Autodesk Inventor part; units mm, degrees
(part 2 of 2)
sketch "Skizze29" plane through (89.6, -2.4765, -33.8) normal (0, 0, -1) x (-1, 0, 0)
  line L0 (43.6, -0.4235) -> (43.6, -0.5235) construction
  line L1 (43.6, -0.5235) -> (49.9, -0.5235) construction
  line L2 (49.9, -0.5235) -> (52.9, 2.4765) construction
  line L3 (52.9, 2.4765) -> (79.4, 2.4765) construction
  line L4 (79.4, 2.4765) -> (79.4, 2.2765) construction
  line L5 (79.4, 2.2765) -> (83.4, 2.2765) construction
  line L6 (83.4, 2.2765) -> (83.4, 7.3765) construction
  line L7 (83.4, 7.3765) -> (49.9, 7.3765) construction
  line L8 (49.9, 7.3765) -> (49.9, 6.7966) construction
  line L9 (49.9, 6.7966) -> (45.4981, 2.3946) construction
  line L10 (45.4981, 2.3946) -> (38.1019, 2.3946) construction
  line L11 (38.1019, 2.3946) -> (33.7, 6.7966) construction
  line L12 (33.7, 6.7966) -> (33.7, 7.3765) construction
  line L13 (33.7, 7.3765) -> (17.2925, 7.3765) construction
  line L14 (17.2925, 7.3765) -> (17.2925, 2.4765) construction
  line L15 (17.2925, 2.4765) -> (31.9, 2.4765) construction
  line L16 (31.9, 2.4765) -> (34.8, -0.4235) construction
  line L17 (34.8, -0.4235) -> (43.6, -0.4235) construction
  line L18 (43.6, -28.4235) -> (34.8, -28.4235) construction
  line L19 (31.9, -31.3235) -> (34.8, -28.4235) construction
  line L20 (17.2925, -31.3235) -> (31.9, -31.3235) construction
  line L21 (17.2925, -31.3235) -> (17.2925, -36.2235) construction
  line L22 (33.7, -36.2235) -> (17.2925, -36.2235) construction
  line L23 (33.7, -36.2235) -> (33.7, -35.6437) construction
  line L24 (38.1019, -31.2417) -> (33.7, -35.6437) construction
  line L25 (45.4981, -31.2417) -> (38.1019, -31.2417) construction
  line L26 (49.9, -35.6437) -> (45.4981, -31.2417) construction
  line L27 (49.9, -35.6437) -> (49.9, -36.2235) construction
  line L28 (83.4, -36.2235) -> (49.9, -36.2235) construction
  line L29 (83.4, -31.1235) -> (83.4, -36.2235) construction
  line L30 (83.4, -31.1235) -> (79.4, -31.1235) construction
  line L31 (79.4, -31.3235) -> (79.4, -31.1235) construction
  line L32 (52.9, -31.3235) -> (79.4, -31.3235) construction
  line L33 (49.9, -28.3235) -> (52.9, -31.3235) construction
  line L34 (43.6, -28.3235) -> (49.9, -28.3235) construction
  line L35 (43.6, -28.3235) -> (43.6, -28.4235) construction
  line L36 (6, -28.8471) -> (0, -28.8471) construction
  line L37 (0, -28.8471) -> (0, -36.2235) construction
  line L38 (0, -36.2235) -> (6, -36.2235) construction
  line L39 (6, -36.2235) -> (6, -28.8471) construction
  line L40 (0, 7.3765) -> (0, 0) construction
  line L41 (0, 0) -> (6, 0) construction
  line L42 (6, 0) -> (6, 7.3765) construction
  line L43 (6, 7.3765) -> (0, 7.3765) construction
  line L44 (0, -28.8471) -> (3.8, -28.8471) construction
  line L45 (3.8, -27.1235) -> (3.8, -28.8471) construction
  line L46 (-4.5838, -27.1235) -> (3.8, -27.1235) construction
  line L47 (-4.5838, -1.7235) -> (-4.5838, -27.1235) construction
  line L48 (-4.5838, -1.7235) -> (3.8, -1.7235) construction
  line L49 (3.8, -1.7235) -> (3.8, 0) construction
  line L50 (3.8, 0) -> (0, 0) construction
  line L51 (0, 0) -> (0, 2.2765) construction
  line L52 (0, 2.2765) -> (-8.2, 2.2765) construction
  line L53 (-8.2, 2.2765) -> (-8.2, -31.1235) construction
  line L54 (0, -31.1235) -> (-8.2, -31.1235) construction
  line L55 (0, -31.1235) -> (0, -28.8471) construction
  line L56 (17.2925, 7.3765) -> (-8.2, 7.3765)
  line L57 (-8.2, 7.3765) -> (-8.2, -36.2235)
  line L58 (-8.2, -36.2235) -> (17.2925, -36.2235)
  line L59 (17.2925, -36.2235) -> (17.2925, 7.3765)
  line L60 (0, -36.2235) -> (6, -36.2235) projected
  point P0 (89.6, 2.4765)
  point P1 (3.8, 2.4765)
  constraints: 8 end point, 2 collinear, 2 parallel, 1 horizontal, 1 perpendicular
extrude "Extrusion29" cut sketch "Skizze29" against normal through all
sketch "Skizze30" plane through (0, 0, 0) normal (0, 0, 1) x (1, 0, 0)
  line L0 (72.3075, -38.7) -> (72.3075, -33.8) construction
  line L1 (57.7, -33.8) -> (72.3075, -33.8) construction
  line L2 (57.7, -33.8) -> (54.8, -30.9) construction
  line L3 (54.8, -30.9) -> (42, -30.9) construction
  line L4 (42, -30.9) -> (42, -30.8) construction
  line L5 (42, -30.8) -> (39.7, -30.8) construction
  line L6 (39.7, -30.8) -> (36.7, -33.8) construction
  line L7 (10.2, -33.8) -> (36.7, -33.8) construction
  line L8 (10.2, -29.4029) -> (10.2, -33.8) construction
  arc A0 (10.2, -4.3971) -> (10.2, -29.4029) centre (14.0958, -16.9) ccw construction
  line L9 (10.2, -4.3971) -> (10.2, 0) construction
  line L10 (10.2, 0) -> (36.7, 0) construction
  line L11 (39.7, -3) -> (36.7, 0) construction
  line L12 (42, -3) -> (39.7, -3) construction
  line L13 (42, -3) -> (42, -2.9) construction
  line L14 (42, -2.9) -> (54.8, -2.9) construction
  line L15 (57.7, 0) -> (54.8, -2.9) construction
  line L16 (57.7, 0) -> (72.3075, 0) construction
  line L17 (72.3075, 0) -> (72.3075, 4.9) construction
  line L18 (72.3075, 4.9) -> (55.9, 4.9) construction
  line L19 (55.9, 4.9) -> (55.9, 4.3201) construction
  line L20 (51.4981, -0.0818) -> (55.9, 4.3201) construction
  line L21 (44.1019, -0.0818) -> (51.4981, -0.0818) construction
  line L22 (39.7, 4.3201) -> (44.1019, -0.0818) construction
  line L23 (39.7, 4.3201) -> (39.7, 4.9) construction
  line L24 (39.7, 4.9) -> (6.2, 4.9) construction
  line L25 (6.2, 4.9) -> (6.2, -0.2) construction
  line L26 (6.2, -0.2) -> (-2, -0.2) construction
  line L27 (-2, -0.2) -> (-2, -33.6) construction
  line L28 (6.2, -33.6) -> (-2, -33.6) construction
  line L29 (6.2, -38.7) -> (6.2, -33.6) construction
  line L30 (39.7, -38.7) -> (6.2, -38.7) construction
  line L31 (39.7, -38.7) -> (39.7, -38.1201) construction
  line L32 (39.7, -38.1201) -> (44.1019, -33.7182) construction
  line L33 (44.1019, -33.7182) -> (51.4981, -33.7182) construction
  line L34 (51.4981, -33.7182) -> (55.9, -38.1201) construction
  line L35 (55.9, -38.1201) -> (55.9, -38.7) construction
  line L36 (72.3075, -38.7) -> (55.9, -38.7) construction
  circle A1 centre (59.1, -36.25) radius 1.4
  line L37 (-16.8615, -16.9) -> (87.169, -16.9) construction
  circle A2 centre (59.1, 2.45) radius 1.4
  line L38 (72.3075, -38.7) -> (72.3075, -33.8) construction
  line L39 (72.3075, -36.25) -> (54.0299, -36.25) construction
  line L40 (51.4981, -33.7182) -> (55.9, -38.1201) construction
  line L41 (57.7, -33.8) -> (54.8, -30.9) construction
  line L42 (57.7, -33.8) -> (57.7, -38.7) construction
  point P0 (0, 0)
  dimension "d149" = 2.8
  constraints: 4 end point, 3 point on line, 2 centre point, 1 horizontal, 1 midpoint, 1 symmetric about line, 1 tangent, 1 vertical, 1 other
  measures "d149" diameter of A1
extrude "Extrusion30" cut sketch "Skizze30" against normal through all
fillet "Rundung1" radius 3 2 edges at (72.3075, -38.7, -3) (72.3075, 4.9, -3)
sketch "Skizze31" plane through (0, 0, 0) normal (0, 0, 1) x (1, 0, 0)
  circle A0 centre (59.1, -36.25) radius 1.4 construction
  circle A1 centre (59.1, 2.45) radius 1.4 construction
  arc A2 (72.3075, 1.9) -> (69.3075, 4.9) centre (69.3075, 1.9) ccw construction
  line L0 (69.3075, 4.9) -> (55.9, 4.9) construction
  line L1 (55.9, 4.9) -> (55.9, 4.3201) construction
  line L2 (51.4981, -0.0818) -> (55.9, 4.3201) construction
  line L3 (44.1019, -0.0818) -> (51.4981, -0.0818) construction
  line L4 (39.7, 4.3201) -> (44.1019, -0.0818) construction
  line L5 (39.7, 4.3201) -> (39.7, 4.9) construction
  line L6 (39.7, 4.9) -> (6.2, 4.9) construction
  line L7 (6.2, 4.9) -> (6.2, -0.2) construction
  line L8 (6.2, -0.2) -> (-2, -0.2) construction
  line L9 (-2, -0.2) -> (-2, -33.6) construction
  line L10 (6.2, -33.6) -> (-2, -33.6) construction
  line L11 (6.2, -38.7) -> (6.2, -33.6) construction
  line L12 (39.7, -38.7) -> (6.2, -38.7) construction
  line L13 (39.7, -38.7) -> (39.7, -38.1201) construction
  line L14 (39.7, -38.1201) -> (44.1019, -33.7182) construction
  line L15 (44.1019, -33.7182) -> (51.4981, -33.7182) construction
  line L16 (51.4981, -33.7182) -> (55.9, -38.1201) construction
  line L17 (55.9, -38.1201) -> (55.9, -38.7) construction
  line L18 (69.3075, -38.7) -> (55.9, -38.7) construction
  arc A3 (69.3075, -38.7) -> (72.3075, -35.7) centre (69.3075, -35.7) ccw construction
  line L19 (72.3075, -35.7) -> (72.3075, -33.8) construction
  line L20 (57.7, -33.8) -> (72.3075, -33.8) construction
  line L21 (57.7, -33.8) -> (54.8, -30.9) construction
  line L22 (54.8, -30.9) -> (42, -30.9) construction
  line L23 (42, -30.9) -> (42, -30.8) construction
  line L24 (42, -30.8) -> (39.7, -30.8) construction
  line L25 (39.7, -30.8) -> (36.7, -33.8) construction
  line L26 (10.2, -33.8) -> (36.7, -33.8) construction
  line L27 (10.2, -29.4029) -> (10.2, -33.8) construction
  arc A4 (10.2, -4.3971) -> (10.2, -29.4029) centre (14.0958, -16.9) ccw construction
  line L28 (10.2, -4.3971) -> (10.2, 0) construction
  line L29 (10.2, 0) -> (36.7, 0) construction
  line L30 (39.7, -3) -> (36.7, 0) construction
  line L31 (42, -3) -> (39.7, -3) construction
  line L32 (42, -3) -> (42, -2.9) construction
  line L33 (42, -2.9) -> (54.8, -2.9) construction
  line L34 (57.7, 0) -> (54.8, -2.9) construction
  line L35 (57.7, 0) -> (72.3075, 0) construction
  line L36 (72.3075, 0) -> (72.3075, 1.9) construction
  line L37 (6.2, 4.9) -> (39.8, 4.9)
  line L38 (39.8, 4.9) -> (39.8, 8)
  line L39 (39.8, 8) -> (6.2, 8)
  line L40 (6.2, 8) -> (6.2, 4.9)
  line L41 (-16.9858, -16.9) -> (87.9146, -16.9) projected
  line L42 (39.7, -38.1201) -> (39.7, -38.7) construction
  line L43 (39.7, -38.7) -> (6.2, -38.7) construction
  line L44 (6.2, -38.7) -> (39.8, -38.7)
  line L45 (39.8, -38.7) -> (39.8, -41.8)
  line L46 (39.8, -41.8) -> (6.2, -41.8)
  line L47 (6.2, -41.8) -> (6.2, -38.7)
  point P0 (0, 0)
  dimension "d153" = 33.6
  dimension "d154" = 49.8
  constraints: 20 end point, 3 symmetric about line, 2 parallel, 1 horizontal, 1 perpendicular
  measures "d153" distance of L38.end L39.end
  measures "d154" distance between parallel lines of L46 L39
extrude "Extrusion31" add sketch "Skizze31" against normal up to surface (6 mm away)
sketch "Sketch32" plane through (0, 0, -6) normal (0, 0, -1) x (-1, 0, 0)
  circle A0 centre (-59.1, -36.25) radius 1.4 projected
  circle A1 centre (-59.1, 2.45) radius 1.4 projected
  arc A2 (-69.3075, 4.9) -> (-72.3075, 1.9) centre (-69.3075, 1.9) ccw projected
  line L0 (-69.3075, 4.9) -> (-55.9, 4.9) projected
  line L1 (-55.9, 4.9) -> (-55.9, 4.3201) projected
  line L2 (-51.4981, -0.0818) -> (-55.9, 4.3201) projected
  line L3 (-44.1019, -0.0818) -> (-51.4981, -0.0818) projected
  line L4 (-39.7, 4.3201) -> (-44.1019, -0.0818) projected
  line L5 (-39.7, 4.3201) -> (-39.7, 4.9) projected
  line L6 (-39.7, 4.9) -> (-39.8, 4.9) projected
  line L7 (-39.8, 4.9) -> (-39.8, 8) projected
  line L8 (-39.8, 8) -> (-6.2, 8) projected
  line L9 (-6.2, 8) -> (-6.2, -0.2) projected
  line L10 (-6.2, -0.2) -> (2, -0.2) projected
  line L11 (2, -0.2) -> (2, -33.6) projected
  line L12 (-6.2, -33.6) -> (2, -33.6) projected
  line L13 (-6.2, -41.8) -> (-6.2, -33.6) projected
  line L14 (-39.8, -41.8) -> (-6.2, -41.8) projected
  line L15 (-39.8, -38.7) -> (-39.8, -41.8) projected
  line L16 (-39.7, -38.7) -> (-39.8, -38.7) projected
  line L17 (-39.7, -38.7) -> (-39.7, -38.1201) projected
  line L18 (-39.7, -38.1201) -> (-44.1019, -33.7182) projected
  line L19 (-44.1019, -33.7182) -> (-51.4981, -33.7182) projected
  line L20 (-51.4981, -33.7182) -> (-55.9, -38.1201) projected
  line L21 (-55.9, -38.1201) -> (-55.9, -38.7) projected
  line L22 (-69.3075, -38.7) -> (-55.9, -38.7) projected
  arc A3 (-72.3075, -35.7) -> (-69.3075, -38.7) centre (-69.3075, -35.7) ccw projected
  line L23 (-72.3075, -35.7) -> (-72.3075, -33.8) projected
  line L24 (-57.7, -33.8) -> (-72.3075, -33.8) projected
  line L25 (-57.7, -33.8) -> (-54.8, -30.9) projected
  line L26 (-54.8, -30.9) -> (-42, -30.9) projected
  line L27 (-42, -30.9) -> (-42, -30.8) projected
  line L28 (-42, -30.8) -> (-39.7, -30.8) projected
  line L29 (-39.7, -30.8) -> (-36.7, -33.8) projected
  line L30 (-10.2, -33.8) -> (-36.7, -33.8) projected
  line L31 (-10.2, -29.4029) -> (-10.2, -33.8) projected
  arc A4 (-10.2, -29.4029) -> (-10.2, -4.3971) centre (-14.0958, -16.9) ccw projected
  line L32 (-10.2, -4.3971) -> (-10.2, 0) projected
  line L33 (-10.2, 0) -> (-36.7, 0) projected
  line L34 (-39.7, -3) -> (-36.7, 0) projected
  line L35 (-42, -3) -> (-39.7, -3) projected
  line L36 (-42, -3) -> (-42, -2.9) projected
  line L37 (-42, -2.9) -> (-54.8, -2.9) projected
  line L38 (-57.7, 0) -> (-54.8, -2.9) projected
  line L39 (-57.7, 0) -> (-72.3075, 0) projected
  line L40 (-72.3075, 0) -> (-72.3075, 1.9) projected
  line L41 (-47.6075, -33.7182) -> (-47.6075, -30.9)
  line L42 (-54.8, -30.9) -> (-42, -30.9) projected
  line L43 (-54.8, -2.9) -> (-46, -2.9) projected
  line L44 (-47.6075, -2.9) -> (-47.6075, -0.0818)
  line L45 (-44.1019, -0.0818) -> (-51.4981, -0.0818) projected
  point P0 (0, 0)
  dimension "d157" = 24.7
  constraints: 6 point on line, 4 end point, 1 perpendicular
  measures "d157" distance between parallel lines of L23 L41
extrude "Extrusion32" add sketch "Sketch32" along normal blind 7 contours A0 | A1 | L0 L1 L2 L3 L44 L37 L38 L39 L40 A2 | L41 L19 L20 L21 L22 A3 L23 L24 L25 L26
sketch "Sketch33" plane through (0, 0, 0) normal (0, 0, 1) x (1, 0, 0)
  circle A0 centre (59.1, -36.25) radius 1.4 projected
  circle A1 centre (59.1, 2.45) radius 1.4 projected
  arc A2 (72.3075, 1.9) -> (69.3075, 4.9) centre (69.3075, 1.9) ccw projected
  line L0 (69.3075, 4.9) -> (55.9, 4.9) projected
  line L1 (55.9, 4.9) -> (55.9, 4.3201) projected
  line L2 (51.4981, -0.0818) -> (55.9, 4.3201) projected
  line L3 (44.1019, -0.0818) -> (51.4981, -0.0818) projected
  line L4 (39.7, 4.3201) -> (44.1019, -0.0818) projected
  line L5 (39.7, 4.3201) -> (39.7, 4.9) projected
  line L6 (39.7, 4.9) -> (39.8, 4.9) projected
  line L7 (39.8, 4.9) -> (39.8, 8) projected
  line L8 (39.8, 8) -> (6.2, 8) projected
  line L9 (6.2, 8) -> (6.2, -0.2) projected
  line L10 (6.2, -0.2) -> (-2, -0.2) projected
  line L11 (-2, -0.2) -> (-2, -33.6) projected
  line L12 (6.2, -33.6) -> (-2, -33.6) projected
  line L13 (6.2, -41.8) -> (6.2, -33.6) projected
  line L14 (39.8, -41.8) -> (6.2, -41.8) projected
  line L15 (39.8, -38.7) -> (39.8, -41.8) projected
  line L16 (39.7, -38.7) -> (39.8, -38.7) projected
  line L17 (39.7, -38.7) -> (39.7, -38.1201) projected
  line L18 (39.7, -38.1201) -> (44.1019, -33.7182) projected
  line L19 (44.1019, -33.7182) -> (51.4981, -33.7182) projected
  line L20 (51.4981, -33.7182) -> (55.9, -38.1201) projected
  line L21 (55.9, -38.1201) -> (55.9, -38.7) projected
  line L22 (69.3075, -38.7) -> (55.9, -38.7) projected
  arc A3 (69.3075, -38.7) -> (72.3075, -35.7) centre (69.3075, -35.7) ccw projected
  line L23 (72.3075, -35.7) -> (72.3075, -33.8) construction
  line L24 (57.7, -33.8) -> (72.3075, -33.8) projected
  line L25 (57.7, -33.8) -> (54.8, -30.9) projected
  line L26 (54.8, -30.9) -> (42, -30.9) projected
  line L27 (42, -30.9) -> (42, -30.8) projected
  line L28 (42, -30.8) -> (39.7, -30.8) projected
  line L29 (39.7, -30.8) -> (36.7, -33.8) projected
  line L30 (10.2, -33.8) -> (36.7, -33.8) projected
  line L31 (10.2, -29.4029) -> (10.2, -33.8) projected
  arc A4 (10.2, -4.3971) -> (10.2, -29.4029) centre (14.0958, -16.9) ccw projected
  line L32 (10.2, -4.3971) -> (10.2, 0) projected
  line L33 (10.2, 0) -> (36.7, 0) projected
  line L34 (39.7, -3) -> (36.7, 0) projected
  line L35 (42, -3) -> (39.7, -3) projected
  line L36 (42, -3) -> (42, -2.9) projected
  line L37 (42, -2.9) -> (54.8, -2.9) projected
  line L38 (57.7, 0) -> (54.8, -2.9) projected
  line L39 (57.7, 0) -> (72.3075, 0) projected
  line L40 (72.3075, 0) -> (72.3075, 1.9) construction
  line L41 (69.3075, 4.9) -> (55.9, 4.9) projected
  line L42 (55.9, 4.9) -> (47.6075, 4.9)
  line L43 (47.6075, 4.9) -> (47.6075, -0.0818)
  line L44 (44.1019, -33.7182) -> (51.4981, -33.7182) projected
  line L45 (47.6075, -33.7182) -> (47.6075, -38.7)
  line L46 (47.6075, -38.7) -> (55.9, -38.7)
  arc A5 (71.7465, -34.4) -> (78.7465, -34.4) centre (75.2465, -34.4) ccw construction
  line L47 (78.7465, -30.4554) -> (78.7465, -34.4) construction
  arc A6 (78.7465, 0.6) -> (71.7465, 0.6) centre (75.2465, 0.6) ccw construction
  line L48 (78.7465, -3.3446) -> (78.7465, 0.6) construction
  point P0 (0, 0)
  dimension "d160" = 24.7
  constraints: 12 end point, 4 point on circle, 4 point on line, 2 centre point, 2 perpendicular, 2 vertical, 1 horizontal, 10 other
  measures "d160" distance between parallel lines of L40 L43
extrude "Extrusion33" add sketch "Sketch33" against normal up to surface (13 mm away)
sketch "Sketch34" plane through (0, 0, -13) normal (0, 0, -1) x (-1, 0, 0)
  line L0 (-47.6075, -38.7) -> (-47.6075, -30.9) projected
  line L1 (-47.6075, -30.9) -> (-54.8, -30.9) projected
  line L2 (-54.8, -30.9) -> (-57.7, -33.8) projected
  line L3 (-57.7, -33.8) -> (-72.3075, -33.8) projected
  line L4 (-72.3075, -33.8) -> (-72.3075, -35.7) projected
  arc A0 (-72.3075, -35.7) -> (-69.3075, -38.7) centre (-69.3075, -35.7) ccw projected
  line L5 (-69.3075, -38.7) -> (-47.6075, -38.7) projected
  line L6 (-72.3075, 1.9) -> (-72.3075, 0) projected
  line L7 (-72.3075, 0) -> (-57.7, 0) projected
  line L8 (-57.7, 0) -> (-54.8, -2.9) projected
  line L9 (-54.8, -2.9) -> (-47.6075, -2.9) projected
  line L10 (-47.6075, -2.9) -> (-47.6075, 4.9) projected
  line L11 (-47.6075, 4.9) -> (-69.3075, 4.9) projected
  arc A1 (-69.3075, 4.9) -> (-72.3075, 1.9) centre (-69.3075, 1.9) ccw projected
  line L12 (-47.6075, -0.0818) -> (-47.6075, -2.9) projected
  line L13 (-47.6075, -30.9) -> (-47.6075, -2.9)
  line L14 (-72.3075, -33.8) -> (-72.3075, 0)
  point P0 (0, 0)
  constraints: 4 end point, 2 vertical
extrude "Extrusion34" add sketch "Sketch34" along normal blind 1
sketch "Sketch35" plane through (0, 0, -14) normal (0, 0, -1) x (-1, 0, 0)
  line L0 (-47.6075, -38.7) -> (-47.6075, 4.9) projected
  line L1 (-47.6075, 4.9) -> (-69.3075, 4.9) projected
  arc A0 (-69.3075, 4.9) -> (-72.3075, 1.9) centre (-69.3075, 1.9) ccw projected
  line L2 (-72.3075, 1.9) -> (-72.3075, -35.7) projected
  arc A1 (-72.3075, -35.7) -> (-69.3075, -38.7) centre (-69.3075, -35.7) ccw projected
  line L3 (-69.3075, -38.7) -> (-47.6075, -38.7) projected
  line L4 (-87.9146, -16.9) -> (16.9858, -16.9) construction
  line L5 (-47.6075, -33.8) -> (-72.3075, -33.8)
  line L6 (-72.3075, 1.9) -> (-72.3075, -35.7) construction
  line L7 (-47.6075, 0) -> (-72.3075, 0)
  line L8 (-47.6075, -33.7182) -> (-47.6075, -38.7) projected
  line L9 (-47.6075, -33.8) -> (-47.6075, -38.7)
  line L10 (-47.6075, -38.7) -> (-69.3075, -38.7)
  arc A2 (-72.3075, -35.7) -> (-69.3075, -38.7) centre (-69.3075, -35.7) ccw projected
  line L11 (-72.3075, -33.8) -> (-72.3075, -35.7)
  line L12 (-47.6075, 4.9) -> (-47.6075, -0.0818) projected
  line L13 (-47.6075, 0) -> (-47.6075, 4.9)
  line L14 (-47.6075, 4.9) -> (-69.3075, 4.9)
  line L15 (-69.263, 4.9) -> (-66.363, 4.9) projected
  line L16 (-72.3075, 0) -> (-72.3075, 1.9) projected
  line L17 (-72.3075, 0) -> (-72.3075, 1.9)
  arc A3 (-69.3075, 4.9) -> (-72.3075, 1.9) centre (-69.3075, 1.9) ccw projected
  arc A4 (-69.3075, 4.9) -> (-72.3075, 1.9) centre (-69.3075, 1.9) ccw
  arc A5 (-72.3075, -35.7) -> (-69.3075, -38.7) centre (-69.3075, -35.7) ccw
  point P0 (0, 0)
  constraints: 16 end point, 4 collinear, 4 point on circle, 2 centre point, 2 concentric, 2 perpendicular, 2 point on line, 2 symmetric about line, 2 tangent, 1 vertical
extrude "Extrusion35" add sketch "Sketch35" along normal blind 8 contours L3 A1 L2 L5 L0 | L2 A0 L1 L0 L7
sketch "Sketch36" plane through (0, 0, -22) normal (0, 0, -1) x (-1, 0, 0)
  line L0 (-47.6075, -33.8) -> (-72.3075, -33.8) projected
  line L1 (-72.3075, -33.8) -> (-72.3075, -35.7) projected
  arc A0 (-72.3075, -35.7) -> (-69.3075, -38.7) centre (-69.3075, -35.7) ccw projected
  line L2 (-72.3075, -33.8) -> (-47.6075, -33.8) projected
  line L3 (-47.6075, -33.8) -> (-47.6075, 0) projected
  line L4 (-47.6075, 0) -> (-72.3075, 0) projected
  line L5 (-72.3075, 0) -> (-72.3075, -33.8) projected
  line L6 (-47.6075, 4.9) -> (-69.3075, 4.9) projected
  arc A1 (-69.3075, 4.9) -> (-72.3075, 1.9) centre (-69.3075, 1.9) ccw projected
  line L7 (-72.3075, 1.9) -> (-72.3075, 0) projected
  line L8 (-72.3075, 0) -> (-47.6075, 0) projected
  line L9 (-47.6075, 0) -> (-47.6075, 4.9) projected
  line L10 (-69.3075, -38.7) -> (-47.6075, -38.7) projected
  line L11 (-47.6075, -38.7) -> (-47.6075, -33.8) projected
  point P0 (0, 0)
extrude "Extrusion36" add sketch "Sketch36" along normal blind 2
sketch "Sketch37" plane through (0, 0, -24) normal (0, 0, -1) x (-1, 0, 0)
  line L0 (-61, -23.9) -> (-71, -23.9) construction
  line L1 (-47.6075, 4.9) -> (-69.3075, 4.9) construction
  arc A0 (-69.3075, 4.9) -> (-72.3075, 1.9) centre (-69.3075, 1.9) ccw construction
  line L2 (-72.3075, 1.9) -> (-72.3075, -35.7) construction
  arc A1 (-72.3075, -35.7) -> (-69.3075, -38.7) centre (-69.3075, -35.7) ccw construction
  line L3 (-87.9146, -16.9) -> (16.9858, -16.9) construction
  circle A2 centre (-67.2465, -16.9) radius 1.7
  line L4 (-47.6075, -38.7) -> (-47.6075, 4.9) projected
  line L5 (-69.3075, -38.7) -> (-47.6075, -38.7) projected
  point P0 (0, 0)
  dimension "d170" = 5.061
  dimension "d171" = 3.4
  constraints: 1 centre point, 1 point on line
  measures "d170" distance from line of L2 A2.centre
  measures "d171" diameter of A2
extrude "Extrusion37" cut sketch "Sketch37" against normal up to surface (11 mm away)
sketch "Sketch38" plane through (0, 0, -13) normal (0, 0, 1) x (1, 0, 0)
  circle A0 centre (67.2465, -16.9) radius 1.7 construction
  line L0 (54.8, -2.9) -> (47.6075, -2.9) construction
  line L1 (47.6075, -30.9) -> (47.6075, -2.9) construction
  line L2 (47.6075, -30.9) -> (54.8, -30.9) construction
  line L3 (54.8, -30.9) -> (57.7, -33.8) construction
  line L4 (57.7, -33.8) -> (72.3075, -33.8) construction
  line L5 (72.3075, 0) -> (72.3075, -33.8) construction
  line L6 (72.3075, 0) -> (57.7, 0) construction
  line L7 (57.7, 0) -> (54.8, -2.9) construction
  circle A1 centre (67.2465, -16.9) radius 2.3
  point P0 (0, 0)
  dimension "d174" = 0.6
  constraints: 1 centre point
  measures "d174" radial gap between concentric circles of A0 A1
extrude "Extrusion38" cut sketch "Sketch38" against normal up to surface (1 mm away)
sketch "Sketch40" plane through (0, 0, 0) normal (0, 0, 1) x (1, 0, 0)
  arc A0 (72.3075, 1.9) -> (69.3075, 4.9) centre (69.3075, 1.9) ccw construction
  line L0 (69.3075, 4.9) -> (47.6075, 4.9) construction
  line L1 (47.6075, 4.9) -> (47.6075, -0.0818) construction
  line L2 (44.1019, -0.0818) -> (47.6075, -0.0818) construction
  line L3 (39.7, 4.3201) -> (44.1019, -0.0818) construction
  line L4 (39.7, 4.3201) -> (39.7, 4.9) construction
  line L5 (39.7, 4.9) -> (39.8, 4.9) construction
  line L6 (39.8, 4.9) -> (39.8, 8) construction
  line L7 (39.8, 8) -> (6.2, 8) construction
  line L8 (6.2, 8) -> (6.2, -0.2) construction
  line L9 (6.2, -0.2) -> (-2, -0.2) construction
  line L10 (-2, -0.2) -> (-2, -33.6) construction
  line L11 (6.2, -33.6) -> (-2, -33.6) construction
  line L12 (6.2, -41.8) -> (6.2, -33.6) construction
  line L13 (39.8, -41.8) -> (6.2, -41.8) construction
  line L14 (39.8, -38.7) -> (39.8, -41.8) construction
  line L15 (39.7, -38.7) -> (39.8, -38.7) construction
  line L16 (39.7, -38.7) -> (39.7, -38.1201) construction
  line L17 (39.7, -38.1201) -> (44.1019, -33.7182) construction
  line L18 (44.1019, -33.7182) -> (47.6075, -33.7182) construction
  line L19 (47.6075, -33.7182) -> (47.6075, -38.7) construction
  line L20 (47.6075, -38.7) -> (69.3075, -38.7) construction
  arc A1 (69.3075, -38.7) -> (72.3075, -35.7) centre (69.3075, -35.7) ccw construction
  line L21 (72.3075, -35.7) -> (72.3075, -33.8) construction
  line L22 (57.7, -33.8) -> (72.3075, -33.8) construction
  line L23 (57.7, -33.8) -> (54.8, -30.9) construction
  line L24 (54.8, -30.9) -> (42, -30.9) construction
  line L25 (42, -30.9) -> (42, -30.8) construction
  line L26 (42, -30.8) -> (39.7, -30.8) construction
  line L27 (39.7, -30.8) -> (36.7, -33.8) construction
  line L28 (10.2, -33.8) -> (36.7, -33.8) construction
  line L29 (10.2, -29.4029) -> (10.2, -33.8) construction
  arc A2 (10.2, -4.3971) -> (10.2, -29.4029) centre (14.0958, -16.9) ccw construction
  line L30 (10.2, -4.3971) -> (10.2, 0) construction
  line L31 (10.2, 0) -> (36.7, 0) construction
  line L32 (39.7, -3) -> (36.7, 0) construction
  line L33 (42, -3) -> (39.7, -3) construction
  line L34 (42, -3) -> (42, -2.9) construction
  line L35 (42, -2.9) -> (54.8, -2.9) construction
  line L36 (57.7, 0) -> (54.8, -2.9) construction
  line L37 (57.7, 0) -> (72.3075, 0) construction
  line L38 (72.3075, 0) -> (72.3075, 1.9) construction
  line L39 (-16.9858, -16.9) -> (87.9146, -16.9) construction
  line L40 (6.2, 8) -> (6.2, 4.2406) construction
  line L41 (6.2, 4.2406) -> (1.7594, -0.2) construction
  line L42 (42, -12.2664) -> (34.1307, -4.3971) construction
  line L43 (1.7594, -0.2) -> (-2, -0.2) construction
  line L44 (6.2, -0.2) -> (-2, -0.2) construction
  line L45 (6.2, 4.2406) -> (1.7594, -0.2)
  line L46 (6.2, 8) -> (6.2, -0.2) projected
  line L47 (1.7594, -0.2) -> (6.2, -0.2)
  line L48 (6.2, -0.2) -> (6.2, 4.2406)
  line L49 (6.2, -33.6) -> (-2, -33.6) construction
  line L50 (6.2, -38.0406) -> (1.7594, -33.6) construction
  line L51 (1.7594, -33.6) -> (-2, -33.6) construction
  line L52 (6.2, -33.6) -> (-2, -33.6) construction
  line L53 (6.2, -38.0406) -> (1.7594, -33.6)
  line L54 (1.7594, -33.6) -> (6.2, -33.6)
  line L55 (6.2, -33.6) -> (6.2, -38.0406)
  point P0 (0, 0)
  point P1 (0, -33.8)
  dimension "d179" = 6.28
  constraints: 26 end point, 5 symmetric about line, 3 perpendicular, 1 collinear, 1 horizontal, 1 point on line
  measures "d179" distance of L40.end L41.end
extrude "Extrusion39" add sketch "Sketch40" against normal up to surface (6 mm away)
sketch "Sketch42" plane through (0, 0, -24) normal (0, 0, -1) x (-1, 0, 0)
  circle A0 centre (-67.2465, -16.9) radius 1.7 construction
  line L0 (-69.3075, -38.7) -> (-47.6075, -38.7) construction
  line L1 (-47.6075, -38.7) -> (-47.6075, 4.9) construction
  line L2 (-47.6075, 4.9) -> (-69.3075, 4.9) construction
  arc A1 (-69.3075, 4.9) -> (-72.3075, 1.9) centre (-69.3075, 1.9) ccw construction
  line L3 (-72.3075, 1.9) -> (-72.3075, -35.7) construction
  arc A2 (-72.3075, -35.7) -> (-69.3075, -38.7) centre (-69.3075, -35.7) ccw construction
  arc A3 (-75.2465, -30.9) -> (-75.2465, -2.9) centre (-75.2465, -16.9) ccw construction
  line L4 (-72.3075, -3.212) -> (-72.3075, -30.588)
  arc A4 (-72.3075, -30.588) -> (-72.3075, -3.212) centre (-75.2465, -16.9) ccw
  point P0 (0, 0)
  constraints: 6 point on circle, 2 centre point, 2 end point, 2 point on line, 4 other
extrude "Extrusion40" cut sketch "Sketch42" against normal up to surface (11 mm away)
sketch "Sketch43" plane through (0, 0, -24) normal (0, 0, -1) x (-1, 0, 0)
  arc A0 (-72.3075, -30.588) -> (-72.3075, -3.212) centre (-75.2465, -16.9) ccw construction
  line L0 (-72.3075, -30.588) -> (-72.3075, -35.7) construction
  arc A1 (-72.3075, -35.7) -> (-69.3075, -38.7) centre (-69.3075, -35.7) ccw construction
  line L1 (-69.3075, -38.7) -> (-47.6075, -38.7) construction
  line L2 (-47.6075, -38.7) -> (-47.6075, 4.9) construction
  line L3 (-47.6075, 4.9) -> (-69.3075, 4.9) construction
  arc A2 (-69.3075, 4.9) -> (-72.3075, 1.9) centre (-69.3075, 1.9) ccw construction
  line L4 (-72.3075, 1.9) -> (-72.3075, -3.212) construction
  line L5 (-78.7465, -30.4554) -> (-78.7465, -34.4) construction
  arc A3 (-78.7465, -34.4) -> (-75.2465, -37.9) centre (-75.2465, -34.4) ccw construction
  arc A4 (-71.7465, 0.6) -> (-78.7465, 0.6) centre (-75.2465, 0.6) ccw construction
  line L6 (-78.7465, -3.3446) -> (-78.7465, 0.6) construction
  line L7 (-72.3075, -3.212) -> (-78.7465, -3.212)
  line L8 (-69.3075, 4.9) -> (-75.7465, 4.9)
  arc A5 (-69.3075, 4.9) -> (-72.3075, 1.9) centre (-69.3075, 1.9) ccw projected
  line L9 (-78.7465, 1.9) -> (-78.7465, -3.212)
  line L10 (-72.3075, -3.212) -> (-72.3075, 1.9)
  line L11 (-72.3075, 1.9) -> (-72.3075, -3.212) projected
  arc A6 (-69.3075, 4.9) -> (-72.3075, 1.9) centre (-69.3075, 1.9) ccw
  arc A7 (-75.7465, 4.9) -> (-78.7465, 1.9) centre (-75.7465, 1.9) ccw
  line L12 (-47.6075, -16.9) -> (-83.9881, -16.9) construction
  line L13 (-72.3075, -30.588) -> (-78.7465, -30.588)
  line L14 (-69.3075, -38.7) -> (-75.7465, -38.7)
  line L15 (-78.7465, -35.7) -> (-78.7465, -30.588)
  line L16 (-72.3075, -30.588) -> (-72.3075, -35.7)
  arc A8 (-72.3075, -35.7) -> (-69.3075, -38.7) centre (-69.3075, -35.7) ccw
  arc A9 (-78.7465, -35.7) -> (-75.7465, -38.7) centre (-75.7465, -35.7) ccw
  circle A10 centre (-75.2465, 0.6) radius 1.4
  circle A11 centre (-75.2465, -34.4) radius 1.4
  point P0 (0, 0)
  dimension "d184" = 3
  dimension "d185" = 2.8
  dimension "d186" = 2.8
  constraints: 22 end point, 12 point on circle, 8 centre point, 5 symmetric about line, 5 tangent, 3 vertical, 2 coincident, 2 horizontal, 1 collinear, 1 concentric, 1 midpoint, 1 perpendicular, 1 point on line, 12 other
  measures "d184" radius of A7
  measures "d185" diameter of A10
  measures "d186" diameter of A11
extrude "Extrusion41" add sketch "Sketch43" against normal up to surface (24 mm away)
sketch "Sketch44" plane through (0, 0, 0) normal (0, 0, 1) x (1, 0, 0)
  circle A0 centre (75.2465, 0.6) radius 1.4 construction
  circle A1 centre (75.2465, -34.4) radius 1.4 construction
  line L0 (75.7465, 4.9) -> (47.6075, 4.9) construction
  line L1 (47.6075, 4.9) -> (47.6075, -0.0818) construction
  line L2 (44.1019, -0.0818) -> (47.6075, -0.0818) construction
  line L3 (39.7, 4.3201) -> (44.1019, -0.0818) construction
  line L4 (39.7, 4.3201) -> (39.7, 4.9) construction
  line L5 (39.7, 4.9) -> (39.8, 4.9) construction
  line L6 (39.8, 4.9) -> (39.8, 8) construction
  line L7 (39.8, 8) -> (6.2, 8) construction
  line L8 (6.2, 8) -> (6.2, 4.2406) construction
  line L9 (6.2, 4.2406) -> (1.7594, -0.2) construction
  line L10 (1.7594, -0.2) -> (-2, -0.2) construction
  line L11 (-2, -0.2) -> (-2, -33.6) construction
  line L12 (1.7594, -33.6) -> (-2, -33.6) construction
  line L13 (1.7594, -33.6) -> (6.2, -38.0406) construction
  line L14 (6.2, -41.8) -> (6.2, -38.0406) construction
  line L15 (39.8, -41.8) -> (6.2, -41.8) construction
  line L16 (39.8, -38.7) -> (39.8, -41.8) construction
  line L17 (39.7, -38.7) -> (39.8, -38.7) construction
  line L18 (39.7, -38.7) -> (39.7, -38.1201) construction
  line L19 (39.7, -38.1201) -> (44.1019, -33.7182) construction
  line L20 (44.1019, -33.7182) -> (47.6075, -33.7182) construction
  line L21 (47.6075, -33.7182) -> (47.6075, -38.7) construction
  line L22 (47.6075, -38.7) -> (75.7465, -38.7) construction
  arc A2 (75.7465, -38.7) -> (78.7465, -35.7) centre (75.7465, -35.7) ccw construction
  line L23 (78.7465, -30.588) -> (78.7465, -35.7) construction
  line L24 (72.3075, -30.588) -> (78.7465, -30.588) construction
  line L25 (72.3075, -33.8) -> (72.3075, -30.588) construction
  line L26 (57.7, -33.8) -> (72.3075, -33.8) construction
  line L27 (57.7, -33.8) -> (54.8, -30.9) construction
  line L28 (54.8, -30.9) -> (42, -30.9) construction
  line L29 (42, -30.9) -> (42, -30.8) construction
  line L30 (42, -30.8) -> (39.7, -30.8) construction
  line L31 (39.7, -30.8) -> (36.7, -33.8) construction
  line L32 (10.2, -33.8) -> (36.7, -33.8) construction
  line L33 (10.2, -29.4029) -> (10.2, -33.8) construction
  arc A3 (10.2, -4.3971) -> (10.2, -29.4029) centre (14.0958, -16.9) ccw construction
  line L34 (10.2, -4.3971) -> (10.2, 0) construction
  line L35 (10.2, 0) -> (36.7, 0) construction
  line L36 (39.7, -3) -> (36.7, 0) construction
  line L37 (42, -3) -> (39.7, -3) construction
  line L38 (42, -3) -> (42, -2.9) construction
  line L39 (42, -2.9) -> (54.8, -2.9) construction
  line L40 (57.7, 0) -> (54.8, -2.9) construction
  line L41 (57.7, 0) -> (72.3075, 0) construction
  line L42 (72.3075, -3.212) -> (72.3075, 0) construction
  line L43 (78.7465, -3.212) -> (72.3075, -3.212) construction
  line L44 (78.7465, 1.9) -> (78.7465, -3.212) construction
  arc A4 (78.7465, 1.9) -> (75.7465, 4.9) centre (75.7465, 1.9) ccw construction
  line L45 (78.7465, -30.588) -> (78.7465, -35.7) projected
  line L46 (72.3075, -3.212) -> (72.3075, 0) projected
  line L47 (78.7465, -30.588) -> (72.3075, -30.588)
  line L48 (72.3075, -30.588) -> (72.3075, -3.212)
  line L49 (72.3075, -3.212) -> (78.7465, -3.212)
  line L50 (78.7465, -3.212) -> (78.7465, -30.588)
  point P0 (0, 0)
  constraints: 8 end point, 2 parallel, 1 horizontal, 1 perpendicular
extrude "Extrusion42" add sketch "Sketch44" against normal up to surface (6 mm away)
sketch "Sketch45" plane through (0, 0, -6) normal (0, 0, -1) x (-1, 0, 0)
  line L0 (-40.7, -12.2681) -> (-40.7, -21.5319) projected
  line L1 (-40.7, -12.2681) -> (-40.7, -10.9664) projected
  line L2 (-42, -12.2664) -> (-40.7, -10.9664) projected
  line L3 (-42, -21.5336) -> (-42, -12.2664) projected
  line L4 (-42, -21.5336) -> (-40.7, -22.8336) projected
  line L5 (-40.7, -21.5319) -> (-40.7, -22.8336) projected
  point P0 (0, 0)
extrude "Extrusion43" add sketch "Sketch45" along normal blind 0.3
ref_plane "Work Plane5" through (6, -38.3, -33.8) normal (0, 0, -1) x (1, 0, 0)
ref_plane "Work Plane6" through (10.2, -29.4, -20.3) normal (0, 0, 1) x (-1, 0, 0)
ref_plane "Work Plane7" through (0, -33.8, -18) normal (0, 0, 1) x (-1, 0, 0)
body "Solid1"
